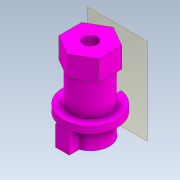
# Autodesk Inventor part: Coupling_0504
Saved by Autodesk Inventor 2022 (Build 260153000, 153)
## iProperties
Created: 2023-03-17
Part Number: Coupling_0504
Material: 一般
Document SubType Name: Modeling
Designer: JOU
Density: 1 g/cm^3
Appearance: 預設
Mass: 1.64153 g
Surface Area: 11.3377 cm^2
Volume: 1.64153 cm^3
Author: JOU
Title: 聯軸器
Autodesk Inventor part; units mm, degrees
ref_plane "YZ Plane" through (0, 0, 0) normal (1, 0, 0) x (0, 1, 0)
ref_plane "XZ Plane" through (0, 0, 0) normal (0, 1, 0) x (-1, 0, 0)
ref_plane "XY Plane" through (0, 0, 0) normal (0, 0, 1) x (1, 0, 0)
sketch "草圖1" plane through (0, 0, 0) normal (0, 1, 0) x (-1, 0, 0)
  circle A0 centre (0, 0) radius 5.5
  dimension "d0" = 11
  constraints: 1 centre point, 1 coincident
  measures "d0" diameter of A0
extrude "擠出1" add sketch "草圖1" along normal blind 18
sketch "草圖2" plane through (0, 18, 0) normal (0, 1, 0) x (1, 0, 0)
  line L0 (5.85, -3.3775) -> (0, -6.755)
  line L1 (0, -6.755) -> (-5.85, -3.3775)
  line L2 (-5.85, -3.3775) -> (-5.85, 3.3775)
  line L3 (-5.85, 3.3775) -> (0, 6.755)
  line L4 (0, 6.755) -> (5.85, 3.3775)
  line L5 (5.85, 3.3775) -> (5.85, -3.3775)
  point P0 (0, 0)
  point P1 (0, 0)
  dimension "d3" = 11.7
  constraints: 12 end point, 1 coincident, 1 vertical, 13 other
  measures "d3" distance between parallel lines of L5 L2
extrude "擠出2" add sketch "草圖2" along normal blind 6
sketch "草圖3" plane through (0, 0, 0) normal (0, -1, 0) x (1, 0, 0)
  circle A0 centre (0, 0) radius 2
  dimension "d6" = 4
  constraints: 1 centre point, 1 coincident
  measures "d6" diameter of A0
extrude "擠出3" cut sketch "草圖3" against normal up to surface (24 mm away)
sketch "草圖14" plane through (0, 0, 0) normal (0, -1, 0) x (1, 0, 0)
  line L0 (-2, 8.1235) -> (2, 8.1235)
  line L1 (2, 8.1235) -> (2, 5.1235)
  line L2 (2, 5.1235) -> (-2, 5.1235)
  line L3 (-2, 5.1235) -> (-2, 8.1235)
  circle A0 centre (0, 0) radius 2 projected
  circle A1 centre (0, 0) radius 5.5 projected
  circle A2 centre (0, 0) radius 5.5 projected
  dimension "d41" = 3
  dimension "d42" = 4
  constraints: 8 end point, 2 parallel, 1 horizontal, 1 perpendicular, 1 point on circle, 2 other
  measures "d41" distance of L0.end L1.end
  measures "d42" distance of L0.start L0.end
extrude "擠出13" add sketch "草圖14" against normal blind 6 contours L0 L1 A1 L3
sketch "草圖15" plane through (0, 6, 0) normal (0, 1, 0) x (1, 0, 0)
  circle A0 centre (0, 0) radius 2 projected
  circle A1 centre (0, 0) radius 8
  dimension "d45" = 16
  constraints: 1 centre point, 1 coincident
  measures "d45" diameter of A1
extrude "擠出14" add sketch "草圖15" along normal blind 2
ref_plane "工作平面3" through (0, 6, -8) normal (0, 0, 1) x (1, 0, 0)
sketch "草圖16" plane through (0, 6, -8) normal (0, 0, 1) x (1, 0, 0)
  line L0 (0, -10.8) -> (0, 22.8) projected
  circle A0 centre (0, 1) radius 1.5
  line L1 (8, 0) -> (-8, 0) projected
  point P0 (0, -6)
  point P1 (2, 0)
  point P2 (-2, 0)
  dimension "d48" = 3
  dimension "d49" = 1
  constraints: 1 centre point, 1 point on line
  measures "d48" diameter of A0
  measures "d49" distance from line of L1 A0.centre
extrude "擠出15" cut sketch "草圖16" along normal blind 8
sketch "草圖17" plane through (0, 6, -8) normal (0, 0, 1) x (1, 0, 0)
  spline S0 degree 6 poles (-1.118, 2) (-1.1527, 1.9612) (-1.1855, 1.9213) (-1.2163, 1.8805) (-1.2451, 1.8389) (-1.272, 1.7965) (-1.316, 1.7207) (-1.3339, 1.6877) (-1.3507, 1.6542) (-1.3664, 1.6205) (-1.3811, 1.5865) (-1.43, 1.463) (-1.4581, 1.3721) (-1.4791, 1.2799) (-1.493, 1.1869) (-1.5, 1.0934) (-1.5, 0.8706) (-1.4866, 0.7413) (-1.4598, 0.613) (-1.4195, 0.4869) (-1.3654, 0.3642) (-1.272, 0.2035) (-1.2451, 0.1611) (-1.2163, 0.1195) (-1.1855, 0.0787) (-1.1527, 0.0388) (-1.118, 0) knots 0 0 0 0 0 0 0 0.13403 0.13403 0.13403 0.13403 0.13403 0.235671 0.235671 0.235671 0.235671 0.235671 0.499988 0.499988 0.499988 0.499988 0.499988 0.865962 0.865962 0.865962 0.865962 0.865962 1 1 1 1 1 1 1 projected
  spline S1 degree 7 poles (1.118, 0) (1.3399, 0.2481) (1.4837, 0.5381) (1.5528, 0.8447) (1.5524, 1.1553) (1.484, 1.4618) (1.3399, 1.7522) (1.118, 2) knots 0 0 0 0 0 0 0 0 1 1 1 1 1 1 1 1 projected
  spline S2 degree 7 poles (-1.118, 0) (-1.0105, -0.1202) (-0.8821, -0.2334) (-0.7334, -0.3331) (-0.5668, -0.4136) (-0.3859, -0.4704) (-0.1952, -0.5) (0.1954, -0.5) (0.3861, -0.4703) (0.5668, -0.4135) (0.7333, -0.3331) (0.8819, -0.2336) (1.0103, -0.1204) (1.118, 0) knots 0 0 0 0 0 0 0 0 0.499689 0.499689 0.499689 0.499689 0.499689 0.499689 1 1 1 1 1 1 1 1 projected
  spline S3 degree 7 poles (1.118, 2) (1.0105, 2.1202) (0.8821, 2.2334) (0.7334, 2.3331) (0.5668, 2.4136) (0.3859, 2.4704) (0.1952, 2.5) (-0.1954, 2.5) (-0.3861, 2.4703) (-0.5668, 2.4135) (-0.7333, 2.3331) (-0.8819, 2.2336) (-1.0103, 2.1204) (-1.118, 2) knots 0 0 0 0 0 0 0 0 0.499689 0.499689 0.499689 0.499689 0.499689 0.499689 1 1 1 1 1 1 1 1 projected
  circle A0 centre (0, 1) radius 1.55
  line L0 (0, -10.8) -> (0, 22.8) projected
  line L1 (8, 2) -> (-8, 2) projected
  point P0 (0, -6)
  point P1 (-1.118, 0)
  point P2 (-1.118, 2)
  point P3 (1.118, 2)
  dimension "d52" = 1
  dimension "d53" = 3.1
  constraints: 1 centre point, 1 point on line, 1 vertical alignment, 5 other
  measures "d52" distance from line of L1 A0.centre
  measures "d53" diameter of A0
extrude "擠出16" cut sketch "草圖17" along normal up to surface contours L1 A0 L0 S3 | S0 S2 L0 A0 L1 | L0 A0 L1 S3 | S2 S1 L1 A0 L0 round surface about axis through (0, 0, 0) along (0, 1, 0) radius 5.5 far side no
sketch "草圖18" plane through (0, 0, 0) normal (0, -1, 0) x (1, 0, 0)
  circle A0 centre (0, 0) radius 5.5
  constraints: 1 centre point, 1 coincident
